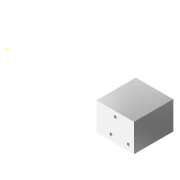
# Autodesk Inventor part: 01_Coolingblock
Saved by Autodesk Inventor 2016 (Build 200138000, 138)
## iProperties
Created: 2016-11-08
Part Number: 01_Coolingblock
Material: Generisch
Document SubType Name: Modeling
Designer: Bene
Density: 1 g/cm^3
Appearance: Chrom - poliert
Author: Bene
Autodesk Inventor part; units mm, degrees
ref_plane "YZ Plane" through (0, 0, 0) normal (1, 0, 0) x (0, 1, 0)
ref_plane "XZ Plane" through (0, 0, 0) normal (0, 1, 0) x (-1, 0, 0)
ref_plane "XY Plane" through (0, 0, 0) normal (0, 0, 1) x (1, 0, 0)
sketch "Skizze1" plane through (0, 0, 0) normal (0, 1, 0) x (-1, 0, 0)
  line L0 (-96.0755, -26.209) -> (-136.0755, -26.209)
  line L1 (-136.0755, -26.209) -> (-136.0755, -56.209)
  line L2 (-136.0755, -56.209) -> (-96.0755, -56.209)
  line L3 (-96.0755, -56.209) -> (-96.0755, -26.209)
  point P0 (0, 0)
  dimension "d0" = 40
  dimension "d1" = 30
  constraints: 8 end point, 2 parallel, 1 horizontal, 1 perpendicular
  measures "d0" distance of L2.end L1.end
  measures "d1" distance of L1.end L0.end
extrude "Extrusion1" add sketch "Skizze1" along normal blind 42
sketch "Skizze2" plane through (96.0755, 0, -26.209) normal (0, 0, 1) x (1, 0, 0)
  point P0 (-96.0755, 0)
sketch "Skizze3" plane through (0, 42, 0) normal (0, 1, 0) x (1, 0, 0)
  circle A0 centre (130.0755, 50.209) radius 1.5
  circle A1 centre (111.5755, 50.209) radius 1.5
  circle A2 centre (116.0755, 31.709) radius 1.5
  line L0 (136.0755, 56.209) -> (96.0755, 56.209) projected
  line L1 (136.0755, 26.209) -> (136.0755, 56.209) projected
  point P0 (0, 0)
  dimension "d4" = 3
  dimension "d5" = 3
  dimension "d6" = 3
  dimension "d7" = 6
  dimension "d8" = 6
  dimension "d9" = 6
  dimension "d10" = 18.5
  dimension "d11" = 18.5
  dimension "d12" = 20
  constraints: 3 centre point
  measures "d4" diameter of A0
  measures "d5" diameter of A1
  measures "d6" diameter of A2
  measures "d7" distance from line of A0.centre L0
  measures "d8" distance from line of A0.centre L1
  measures "d9" distance from line of L0 A1.centre
  measures "d10" distance of A0.centre A1.centre
  measures "d11" vertical distance of A2.centre A1.centre
  measures "d12" distance from line of A2.centre L1
extrude "Extrusion2" cut sketch "Skizze3" against normal through all
